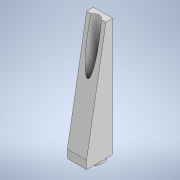
# Autodesk Inventor part: rpi_stand
Saved by Autodesk Inventor 2020 (Build 240168000, 168)
## iProperties
Created: 2020-12-18
Part Number: rpi_stand
Material: Generic
Document SubType Name: Modeling
Designer: agupta40
Density: 1 g/cm^3
Appearance: Default
Author: agupta40
Autodesk Inventor part; units mm, degrees
ref_plane "YZ Plane" through (0, 0, 0) normal (1, 0, 0) x (0, 1, 0)
ref_plane "XZ Plane" through (0, 0, 0) normal (0, 1, 0) x (-1, 0, 0)
ref_plane "XY Plane" through (0, 0, 0) normal (0, 0, 1) x (1, 0, 0)
sketch "Sketch1" plane through (0, 0, 0) normal (1, 0, 0) x (0, 1, 0)
  line L0 (0, 0) -> (0, 9.5)
  line L1 (0, 9.5) -> (3, 9.5)
  line L2 (3, 9.5) -> (43, 2.4469)
  line L3 (43, 2.4469) -> (43, 0)
  line L4 (43, 0) -> (0, 0)
  dimension "d0" = 9.5
  dimension "d1" = 170
  dimension "d2" = 40
  dimension "d4" = 3
  constraints: 10 end point, 2 perpendicular, 1 parallel, 1 vertical
  measures "d0" distance of L0.start L0.end
  measures "d1" angle of L1 L2
  measures "d2" horizontal distance of L1.end L2.end
  measures "d4" distance of L0.end L1.end
extrude "Extrusion1" add sketch "Sketch1" along normal blind 7
sketch "Sketch2" plane through (0, 0, 0) normal (0, -1, 0) x (1, 0, 0)
  circle A0 centre (3.5, 3.5) radius 3.5
  line L0 (0, 9.5) -> (0, 0) projected
  line L1 (7, 9.5) -> (7, 0) projected
  line L2 (0, 0) -> (7, 0) projected
  circle A1 centre (3.5, 3.5) radius 2.875
  circle A2 centre (3.5, 3.5) radius 1.375
  dimension "d7" = 5.75
  dimension "d8" = 2.75
  constraints: 3 centre point, 3 tangent, 2 coincident
  measures "d7" diameter of A1
  measures "d8" diameter of A2
extrude "Extrusion2" cut sketch "Sketch2" against normal through all contours A2
extrude "Extrusion3" cut sketch "Sketch2" against normal blind 4.25 contours A1
extrude "Extrusion4" add sketch "Sketch2" along normal blind 1 contours A0
sketch "Sketch3" plane through (0, 43, 2.4469) normal (0, 1, 0) x (1, 0, 0)
  arc A0 (4.3841, 0) -> (2.6159, 0) centre (3.5, -1.0531) ccw projected
  circle A1 centre (3.5, -1.0531) radius 2.125
  point P0 (0, 2.4469)
  dimension "d15" = 4.25
  constraints: 1 centre point, 1 coincident
  measures "d15" diameter of A1
extrude "Extrusion5" cut sketch "Sketch3" against normal blind 40
body "Solid1"
